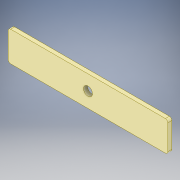
# Autodesk Inventor part: Stress Tester Sample
Saved by Autodesk Inventor 2017 (Build 210142000, 142)
## iProperties
Created: 2017-01-27
Part Number: Stress Tester Sample
Material: Generic
Document SubType Name: Modeling
Designer: kurti
Density: 1 g/cm^3
Appearance: Nylon 6
Author: kurti
Autodesk Inventor part; units mm, degrees
ref_plane "YZ Plane" through (0, 0, 0) normal (1, 0, 0) x (0, 1, 0)
ref_plane "XZ Plane" through (0, 0, 0) normal (0, 1, 0) x (-1, 0, 0)
ref_plane "XY Plane" through (0, 0, 0) normal (0, 0, 1) x (1, 0, 0)
sketch "Sketch1" plane through (0, 0, 0) normal (0, 0, 1) x (1, 0, 0)
  line L0 (-101.6, -19.05) -> (101.6, -19.05)
  line L1 (101.6, -19.05) -> (101.6, 19.05)
  line L2 (101.6, 19.05) -> (-101.6, 19.05)
  line L3 (-101.6, 19.05) -> (-101.6, -19.05)
  line L4 (-101.6, -19.05) -> (101.6, 19.05) construction
  line L5 (101.6, -19.05) -> (-101.6, 19.05) construction
  circle A0 centre (0, 0) radius 5.715
  dimension "d0" = 203.2
  dimension "d1" = 38.1
  dimension "d2" = 11.43
  constraints: 12 end point, 2 midpoint, 2 parallel, 1 centre point, 1 coincident, 1 horizontal, 1 perpendicular
  measures "d0" distance of L2.end L1.end
  measures "d1" distance of L1.end L0.end
  measures "d2" diameter of A0
extrude "Extrusion1" add sketch "Sketch1" along normal blind 5.08
fillet "Fillet1" radius 3.175 4 edges at (-101.6, 19.05, 2.54) (-101.6, -19.05, 2.54) (101.6, 19.05, 2.54) (101.6, -19.05, 2.54)
body "Solid1"
